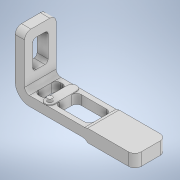
# Autodesk Inventor part: LBody
Saved by Autodesk Inventor 2020.2 (Build 242310000, 310)
## iProperties
Created: 2020-03-03
Part Number: LBody
Material: Generic
Document SubType Name: Modeling
Designer: Kjell
Density: 1 g/cm^3
Appearance: Default
Author: Kjell
Autodesk Inventor part; units mm, degrees
ref_plane "YZ Plane" through (0, 0, 0) normal (1, 0, 0) x (0, 1, 0)
ref_plane "XZ Plane" through (0, 0, 0) normal (0, 1, 0) x (-1, 0, 0)
ref_plane "XY Plane" through (0, 0, 0) normal (0, 0, 1) x (1, 0, 0)
derived "master_sketch.ipt"
sketch "BottomPlateMainDim" plane through (0, 0, 0) normal (0, 0, 1) x (1, 0, 0)
  circle A0 centre (0, 0) radius 3
  circle A1 centre (-42, -7) radius 1.5
  line L0 (-55, 11) -> (-55, -11)
  line L1 (0, 0) -> (-55, 0)
  line L2 (-15, 10) -> (15, 10)
  line L3 (15, 10) -> (15, -10)
  line L4 (15, -10) -> (-15, -10)
  line L5 (-15, -10) -> (-15, 10)
  line L6 (-15, 10) -> (15, -10) construction
  line L7 (15, 10) -> (-15, -10) construction
sketch "FronProfile" plane through (0, 0, 0) normal (0, 1, 0) x (-1, 0, 0)
  line L0 (-15, 0) -> (-15, 8)
  line L1 (-15, 8) -> (15, 8)
  line L2 (15, 8) -> (15, 0)
  line L3 (15, 7.5) -> (52, 7.5)
  line L4 (15, 1.5) -> (52, 1.5)
  line L5 (15, 0) -> (-15, 0)
  line L6 (55, 10.5) -> (55, 14.7599) construction
  line L7 (55, 10.5) -> (55, 40.5)
  line L8 (55, 40.5) -> (61, 40.5)
  line L9 (61, 40.5) -> (61, 10.5)
  arc A0 (52, 7.5) -> (55, 10.5) centre (52, 10.5) ccw
  arc A1 (52, 1.5) -> (61, 10.5) centre (52, 10.5) ccw
  point P0 (0, 0)
  point P1 (15, 0)
  point P2 (55, 0)
  point P3 (55, 0)
  point P4 (55, 0)
sketch "DovetailWeld" plane through (0, 0, 0) normal (0, 0, 1) x (1, 0, 0)
  line L0 (12, 8) -> (-12, 8)
  line L1 (-12, 8) -> (-12, -8)
  line L2 (-12, -8) -> (12, -8)
  line L3 (12, -8) -> (12, 8)
  line L4 (12, 8) -> (-12, -8) construction
  line L5 (-12, 8) -> (12, -8) construction
  point P0 (0, 0)
extrude "Extrusion1" add sketch "FronProfile" along normal mid plane 20
fillet "Fillet1" radius 4 1 edges at (-15, 0, 7.5)
fillet "Fillet2" radius 4 1 edges at (-15, 0, 1.5)
sketch "Sketch3" plane through (-52, -10, 7.5) normal (0, 0, 1) x (1, 0, 0)
  line L0 (0, 20) -> (35.0635, 20) projected
  circle A0 centre (10, 3) radius 1.5 projected
  line L1 (10, 3) -> (10, 17) construction
  line L2 (13, 3) -> (13, 17)
  line L3 (7, 17) -> (7, 3)
  arc A1 (7, 3) -> (13, 3) centre (10, 3) ccw
  arc A2 (13, 17) -> (7, 17) centre (10, 17) ccw
  point P0 (52, 10)
  point P1 (10, 10)
  dimension "d5" = 6
  constraints: 8 end point, 5 tangent, 4 point on circle, 2 centre point, 1 midpoint, 1 parallel, 1 vertical
  measures "d5" diameter of A2
extrude "Extrusion2" add sketch "Sketch3" along normal blind 2.5 contours A0
extrude "Extrusion3" add sketch "Sketch3" along normal up to surface (0.5 mm away)
sketch "Sketch4" plane through (-16.9365, -10, 7.5) normal (0, 0, 1) x (1, 0, 0)
  line L0 (0, 0) -> (-25.0635, 0) projected
  line L1 (0, 20) -> (0, 0) projected
  line L2 (-25.0635, 20) -> (0, 20) projected
  line L3 (-22.0635, 17) -> (-22.0635, 3) projected
  line L4 (-25.0635, 0) -> (-35.0635, 0) projected
  line L5 (-35.0635, 0) -> (-35.0635, 20) projected
  line L6 (-28.0635, 3) -> (-28.0635, 17) projected
  line L7 (-22.0635, 17) -> (-22.0635, 3) projected
  line L8 (-19.0635, 17) -> (-3, 17)
  line L9 (0, 14) -> (0, 6)
  line L10 (-3, 3) -> (-19.0635, 3)
  line L11 (-22.0635, 6) -> (-22.0635, 14)
  arc A0 (-19.0635, 17) -> (-22.0635, 14) centre (-19.0635, 14) ccw
  arc A1 (0, 14) -> (-3, 17) centre (-3, 14) ccw
  arc A2 (-3, 3) -> (0, 6) centre (-3, 6) ccw
  arc A3 (-22.0635, 6) -> (-19.0635, 3) centre (-19.0635, 6) ccw
  line L12 (-32.0635, 17) -> (-31.0635, 17)
  line L13 (-28.0635, 14) -> (-28.0635, 6)
  line L14 (-31.0635, 3) -> (-32.0635, 3)
  line L15 (-35.0635, 6) -> (-35.0635, 14)
  arc A4 (-32.0635, 17) -> (-35.0635, 14) centre (-32.0635, 14) ccw
  arc A5 (-28.0635, 14) -> (-31.0635, 17) centre (-31.0635, 14) ccw
  arc A6 (-31.0635, 3) -> (-28.0635, 6) centre (-31.0635, 6) ccw
  arc A7 (-35.0635, 6) -> (-32.0635, 3) centre (-32.0635, 6) ccw
  point P0 (16.9365, 10)
  dimension "Wall" = 3
  dimension "d11" = 3
  dimension "d12" = 3
  dimension "d13" = 3
  constraints: 16 end point, 16 point on circle, 16 tangent, 8 centre point, 6 collinear, 6 equal radius, 4 parallel, 2 horizontal, 2 perpendicular
  measures "Wall" distance between parallel lines of L2 L8
  measures "d11" distance between parallel lines of L10 L0
  measures "d12" radius of A0
  measures "d13" radius of A4
extrude "Extrusion4" cut sketch "Sketch4" against normal through all
fillet "Fillet3" radius 4 4 edges at (15, -10, 4) (15, 10, 4) (-58, -10, 40.5) (-58, 10, 40.5)
sketch "Sketch5" plane through (-15, -10, 0) normal (0, 0, -1) x (-1, 0, 0)
  circle A0 centre (-15, 10) radius 6.5
  line L0 (-3, 2) -> (-27, 2) projected
  line L1 (-3, 18) -> (-3, 2) projected
  line L2 (-27, 18) -> (-3, 18) projected
  line L3 (-27, 2) -> (-27, 18) projected
  dimension "d17" = 13
  constraints: 1 centre point, 1 coincident
  measures "d17" diameter of A0
extrude "Extrusion5" cut sketch "Sketch5" against normal blind 3 contours A0
extrude "Extrusion6" add sketch "Sketch5" along normal blind 1
fillet "Fillet4" radius 2 4 edges at (12, 8, -0.5) (12, -8, -0.5) (-12, 8, -0.5) (-12, -8, -0.5)
offset faces "Size1" outward -0.1 faces at (3.3333, -8, -0.3333) (11.3603, -7.4661, -0.3333) (-11.7321, -7, -0.3333) (-12, -2, -0.3333) (12, 2, -0.3333) (11.3603, 7.4661, -0.3333) (-3.3333, 8, -0.3333) (-11.4661, 7.3603, -0.3333)
sketch "Sketch7" plane through (-61, -10, 10.5) normal (-1, 0, 0) x (0, 0, 1)
  arc A0 (30, 16) -> (26, 20) centre (26, 16) ccw projected
  line L0 (0, 20) -> (26, 20) projected
  line L1 (0, 0) -> (0, 20) projected
  line L2 (26, 0) -> (0, 0) projected
  arc A1 (26, 0) -> (30, 4) centre (26, 4) ccw projected
  line L3 (30, 4) -> (30, 16) projected
  line L4 (30, 28.6746) -> (30, -6.0887) construction
  line L5 (0, 29.7861) -> (0, -9.1031) construction
  line L6 (15, 26.3494) -> (15, -6.0887) construction
  line L7 (32.0134, 20) -> (-3.6803, 20) construction
  line L8 (32.6465, 0) -> (-2.8663, 0) construction
  line L9 (31.5009, 10) -> (-2.0222, 10) construction
  line L10 (27, 18) -> (3, 18)
  line L11 (3, 18) -> (3, 2)
  line L12 (3, 2) -> (27, 2)
  line L13 (27, 2) -> (27, 18)
  line L14 (27, 18) -> (3, 2) construction
  line L15 (3, 18) -> (27, 2) construction
  point P0 (-10.5, 10)
  point P1 (15, 10)
  dimension "d24" = 24
  dimension "d25" = 16
  constraints: 24 end point, 4 collinear, 4 horizontal, 3 vertical, 2 midpoint, 2 parallel, 2 point on line, 1 perpendicular, 2 other
  measures "d24" distance of L12.end L11.end
  measures "d25" distance of L11.end L10.end
extrude "Extrusion7" add sketch "Sketch7" along normal blind 1 contours L13 L12 L11 L10
fillet "Fillet5" radius 2 4 edges at (-61.5, -8, 13.5) (-61.5, -8, 37.5) (-61.5, 8, 37.5) (-61.5, 8, 13.5)
offset faces "Size2" outward -0.1 faces at (-61.3333, 8, 28.8333) (-61.6667, 6.2981, 13.5223) (-61.3333, 2, 13.5) (-61.3333, -6.2981, 13.5223) (-61.3333, -8, 22.1667) (-61.3333, -7.7321, 36.5) (-61.3333, -2, 37.5) (-61.3333, 7.7321, 36.5)
sketch "Sketch8" plane through (-62, -10, 10.5) normal (-1, 0, 0) x (0, 0, 1)
  arc A0 (5, 17.9) -> (3.1, 16) centre (5, 16) ccw projected
  line L0 (3.1, 16) -> (3.1, 4) projected
  arc A1 (3.1, 4) -> (5, 2.1) centre (5, 4) ccw projected
  line L1 (5, 2.1) -> (25, 2.1) projected
  arc A2 (25, 2.1) -> (26.9, 4) centre (25, 4) ccw projected
  line L2 (26.9, 4) -> (26.9, 16) projected
  arc A3 (26.9, 16) -> (25, 17.9) centre (25, 16) ccw projected
  line L3 (25, 17.9) -> (5, 17.9) projected
  line L4 (23.9, 12.9) -> (23.9, 7.1)
  line L5 (21.9, 5.1) -> (8.1, 5.1)
  line L6 (6.1, 7.1) -> (6.1, 12.9)
  line L7 (8.1, 14.9) -> (21.9, 14.9)
  arc A4 (23.9, 12.9) -> (21.9, 14.9) centre (21.9, 12.9) ccw
  arc A5 (21.9, 5.1) -> (23.9, 7.1) centre (21.9, 7.1) ccw
  arc A6 (6.1, 7.1) -> (8.1, 5.1) centre (8.1, 7.1) ccw
  arc A7 (8.1, 14.9) -> (6.1, 12.9) centre (8.1, 12.9) ccw
  point P0 (-10.5, 10)
  dimension "d30" = 3
  dimension "d31" = 2
  constraints: 8 end point, 8 point on circle, 8 tangent, 4 centre point, 3 equal radius, 3 other
  measures "d30" distance between parallel lines of L2 L4
  measures "d31" radius of A4
extrude "Extrusion8" cut sketch "Sketch8" against normal through all contours L4 A5 L5 A6 L6 A7 L7 A4
equation "\"d11\" = Wall"
body "Solid1"
